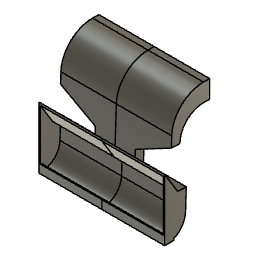
Goal_Chute (Autodesk Fusion 360 design; units mm, degrees)
Autodesk Fusion 360 part; units mm, degrees
note: some values were not read from the file. Set by a fixed rule: which sketch regions a step uses.
sketch "Sketch1" plane through (0, 0, 0) normal (0, 1, 0) x (1, 0, 0) in component "Front Board"
  line L0 (-457.2, -152.4) -> (457.2, -152.4)
  line L1 (457.2, -152.4) -> (457.2, 152.4)
  line L2 (457.2, 152.4) -> (-457.2, 152.4)
  line L3 (-457.2, 152.4) -> (-457.2, -152.4)
  line L4 (-127, -53.975) -> (127, -53.975)
  line L5 (127, -53.975) -> (127, 50.8)
  line L6 (127, 50.8) -> (-127, 50.8)
  line L7 (-127, 50.8) -> (-127, -53.975)
  dimension "d10" = 914.4
  dimension "d11" = 304.8
  dimension "d14" = 254
  dimension "d15" = 104.775
  dimension "d16" = 98.425
  dimension "d189" = 152.4
  dimension "d190" = 127
  dimension "d258" = 457.2
  constraint horizontal L0
  constraint vertical L1
  constraint horizontal L2
  constraint vertical L3
  constraint horizontal L4
  constraint vertical L5
  constraint horizontal L6
  constraint vertical L7
  measures "d10" distance of L0.start L0.end
  measures "d11" distance of L0.start L2.end
  measures "d14" distance of L4.start L4.end
  measures "d15" distance of L4.start L6.end
  measures "d16" distance of L0 L4
  measures "d189" distance of origin L0
  measures "d190" distance of origin L5
  measures "d258" distance of origin L3
extrude "Extrude1" add sketch "Sketch1" against normal blind 12.7 makes body 1 in component "Front Board"
sketch "Sketch1 (2)" plane through (0, 0, 0) normal (0, 1, 0) x (1, 0, 0) in component "Back Board"
  line L0 (457.2, -110.3312) -> (-457.2, -110.3312)
  line L1 (-457.2, -110.3312) -> (-457.2, 110.3312)
  line L2 (-457.2, 110.3312) -> (457.2, 110.3312)
  line L3 (457.2, 110.3312) -> (457.2, -110.3312)
  line L4 (114.3, -110.3312) -> (114.3, -89.6938)
  line L5 (114.3, -89.6938) -> (-114.3, -89.6938)
  line L6 (-114.3, -89.6938) -> (-114.3, -110.3312)
  dimension "d20" = 914.4
  dimension "d21" = 220.6625
  dimension "d22" = 110.3313
  dimension "d23" = 457.2
  dimension "d24" = 200.025
  dimension "d25" = 228.6
  dimension "d26" = 114.3
  constraint horizontal L0
  constraint vertical L1
  constraint horizontal L2
  constraint vertical L3
  constraint coincident L0 L4.start
  constraint perpendicular L0 L4
  constraint perpendicular L4 L5
  constraint coincident L0 L6.end
  constraint perpendicular L0 L6
  measures "d20" distance of L0.start L0.end
  measures "d21" distance of L0.start L2.end
  measures "d22" distance of origin L0
  measures "d23" distance of origin L3
  measures "d24" distance of L2 L5
  measures "d25" distance of L4.end L5.end
  measures "d26" distance of origin L4
extrude "Extrude1'" add sketch "Sketch1 (2)" against normal blind 12.7 separate body contours L0 L1 L2 L3 L4 L5 L6 makes body 2 in component "Back Board"
sketch "Sketch2" plane through (0, 0, 0) normal (1, 0, 0) x (0, 1, 0) in component "Chute"
  line L0 (0, -50.8) -> (2.54, -50.8)
  line L1 (2.54, -50.8) -> (2.54, -65.7225)
  arc A0 (2.54, -65.7225) -> (40.64, -28.8941) centre (2.5612, -27.6225) ccw
  line L2 (40.64, -28.8941) -> (44.45, 85.198)
  arc A1 (95.25, 134.3025) -> (44.45, 85.198) centre (95.2217, 83.5025) ccw
  line L3 (0, -50.8) -> (0, -68.2625)
  arc A2 (95.25, 166.0525) -> (32.4145, 105.3077) centre (95.2217, 103.2103) ccw
  arc A3 (2.54, -68.2625) -> (43.1786, -28.9789) centre (2.5612, -27.6225) ccw
  arc A4 (95.25, 131.7625) -> (46.9886, 85.1132) centre (95.2217, 83.5025) ccw
  line L4 (95.25, 134.3025) -> (95.25, 131.7625)
  line L5 (46.9886, 85.1132) -> (43.1786, -28.9789)
  line L6 (32.4145, 105.3077) -> (29.4039, 15.1538)
  line L7 (95.25, 166.0525) -> (95.25, 168.5925)
  arc A5 (95.25, 168.5925) -> (29.8759, 105.3924) centre (95.2217, 103.2103) ccw
  line L8 (0, 53.975) -> (0, 58.815)
  line L9 (29.8759, 105.3924) -> (26.8653, 15.2386)
  line L10 (46.9886, 85.1132) -> (44.45, 85.198)
  line L11 (31.7571, 85.6219) -> (29.2185, 85.7066)
  line L12 (31.7571, 85.6219) -> (44.45, 85.198)
  line L13 (95.25, 166.0525) -> (95.25, 134.3025)
  line L14 (0, 53.975) -> (0, -50.8)
  line L15 (95.25, 134.3025) -> (107.95, 134.3025)
  line L16 (107.95, 131.7625) -> (107.95, 134.3025)
  line L17 (95.25, 131.7625) -> (107.95, 131.7625)
  line L18 (95.25, 168.5925) -> (107.95, 168.5925)
  line L19 (107.95, 168.5925) -> (107.95, 166.0525)
  line L20 (107.95, 166.0525) -> (95.25, 166.0525)
  line L21 (92.71, 131.6971) -> (92.71, 168.5442)
  line L22 (42.012, 12.1914) -> (26.7805, 12.7)
  line L23 (42.012, 12.1914) -> (44.5506, 12.1066)
  line L24 (42.0968, 14.7299) -> (44.6354, 14.6452)
  line L25 (29.4039, 15.1538) -> (29.3191, 12.6152)
  line L26 (26.8653, 15.2386) -> (26.7805, 12.7)
  line L27 (42.0968, 14.7299) -> (29.4039, 15.1538)
  line L28 (26.8653, 15.2386) -> (29.4039, 15.1538)
  line L29 (0, 58.815) -> (26.8653, 15.2386)
  line L30 (26.7805, 12.7) -> (25.4184, 12.7455)
  line L31 (25.4184, 12.7455) -> (0, 53.975)
  line L32 (19.05, -61.9697) -> (19.05, -64.7672)
  line L33 (0, -68.2625) -> (2.54, -68.2625)
  line L34 (2.54, -68.2625) -> (19.05, -68.2625)
  line L35 (19.05, -68.2625) -> (19.05, -64.7672)
  line L36 (2.54, -65.7225) -> (0, -65.7225)
  line L37 (2.54, -65.7225) -> (19.05, -65.7225)
  line L38 (95.25, 144.4625) -> (92.71, 144.4625)
  line L39 (107.95, 166.0525) -> (107.95, 134.3025)
  point P0 (0, -50.8)
  point P1 (0, 53.975)
  point P2 (95.25, 131.7625)
  point P3 (107.95, 152.4)
  point P4 (95.25, -68.2625)
  dimension "d252" = 2.54
  dimension "d254" = 38.1
  dimension "d256" = 38.1
  dimension "d260" = 50.8
  dimension "d261" = 50.8
  dimension "d272" = 2.54
  dimension "d273" = 2.54
  dimension "d275" = 48.26
  dimension "d276" = 12.7
  dimension "d277" = 2.54
  dimension "d280" = 2.54
  dimension "d281" = 65.3822
  dimension "d282" = 62.8422
  dimension "d324" = 2.54
  dimension "d327" = 40.64
  dimension "d341" = 63.5
  dimension "d346" = 2.54
  dimension "d347" = 2.54
  dimension "d352" = 19.05
  dimension "d371" = 31.75
  dimension "d372" = 12.7
  constraint horizontal L0
  constraint perpendicular L0 L1
  constraint coincident P0 L0.start
  constraint tangent A0 L2
  constraint perpendicular L0 L3
  constraint tangent L2 A1
  constraint vertical A1.centre A2.centre
  constraint vertical L4
  constraint equal L2 L5
  constraint parallel L2 L5
  constraint tangent A4 L5
  constraint tangent A2 L6
  constraint parallel L2 L6
  constraint vertical L7
  constraint coincident P1 L8.start
  constraint vertical L8
  constraint parallel L6 L9
  constraint tangent A5 L9
  constraint tangent A3 L5
  constraint coincident L6 L11.start
  constraint coincident L9 L11.end
  constraint perpendicular L9 L11
  constraint collinear L10 L11
  constraint coincident L2 L22.start
  constraint coincident P2 A4.start
  constraint perpendicular L13 L15
  constraint perpendicular L16 L17
  constraint perpendicular L15 L16
  constraint perpendicular L18 L19
  constraint perpendicular L19 L20
  constraint perpendicular L7 L18
  constraint coincident A2.start L7.start
  constraint vertical L15.end L18.end
  constraint coincident A4 L21.start
  constraint coincident A5 L21.end
  constraint vertical L21
  constraint coincident L2 L24.start
  constraint coincident L9.end L26.start
  constraint coincident L5 L23.end
  constraint coincident L5 L24.end
  constraint coincident L22 L26.end
  constraint parallel L9 L26
  constraint parallel L6 L25
  constraint coincident L22 L25.end
  constraint parallel L22 L23
  constraint parallel L27 L28
  constraint parallel L24 L27
  constraint parallel L29 L31
  constraint parallel L22 L30
  constraint perpendicular L2 L22
  constraint parallel L22 L27
  constraint coincident A0 L32.start
  constraint coincident A3 L32.end
  constraint vertical L32
  constraint perpendicular L3 L33
  constraint vertical L1.end A3.start
  constraint coincident A3.start L33.end
  constraint horizontal L34
  constraint vertical L35
  constraint horizontal L3.end P4
  constraint coincident L3 L36.end
  constraint perpendicular L3 L36
  constraint coincident L32 L37.end
  constraint perpendicular L1 L37
  constraint vertical L19.end P3
  constraint coincident L13 L38.start
  constraint coincident L21 L38.end
  constraint perpendicular L21 L38
  measures "d252" distance of P0 L0.end
  measures "d254" radius of A0
  measures "d256" horizontal distance of L1.end A0.end
  measures "d260" radius of A1
  measures "d261" horizontal distance of A1.start L2.end
  measures "d272" distance of A1.start P2
  measures "d273" distance of L2 L5
  measures "d275" radius of A4
  measures "d276" distance of L2 L6
  measures "d277" distance of A2.start L7.end
  measures "d280" distance of L6 L9
  measures "d281" radius of A5
  measures "d282" radius of A2
  measures "d324" distance of L13 L21
  measures "d327" radius of A3
  measures "d341" vertical distance of P0 L22.end
  measures "d346" distance of L29 L31
  measures "d347" distance of L22 L27
  measures "d352" distance of L3 L32
  measures "d371" distance of L15.end L19.end
  measures "d372" distance of P2 L38.start
extrude "Extrude3" add sketch "Sketch2" along normal blind 2.54 separate body contours A2 L6 A5 L9 L11 L21 | A1 A2 L6 L12 L21 | A2 L7 A5 L21 | A1 A4 L10 L21 | L7 L18 L19 L20 | A2 L13 L21 L38 | A1 L13 L21 L38 | A1 A4 L4 L21 | L13 L15 L20 L39 | L4 L15 L16 L17 makes body 3 in component "Chute"
extrude "Extrude4" add sketch "Sketch2" along normal blind 114.3 contours A2 L6 A5 L9 L11 L21 | A2 L7 A5 L21 | A1 A4 L10 L21 | L7 L18 L19 L20 | A1 A4 L4 L21 | L4 L15 L16 L17 bodies 3 in component "Chute"
extrude "Extrude5" add sketch "Sketch2" against normal blind 2.54 from surface at -12.7 separate body contours A0 A3 L32 L37 | L0 L1 A0 L2 L14 L22 L30 L31 | L0 L1 L3 L36 | L3 A3 L33 L36 L37 | L8 L26 L29 L30 L31 | A0 L2 A3 L5 L23 L32 | L22 L25 L26 L28 | L2 L22 L25 L27 | L2 L5 L23 L24 makes body 4 in component "Chute"
extrude "Extrude6" add sketch "Sketch2" along normal blind 88.9 from surface at -12.7 contours A0 A3 L32 L37 | L0 L1 L3 L36 | L3 A3 L33 L36 L37 | L8 L26 L29 L30 L31 | A0 L2 A3 L5 L23 L32 | L22 L25 L26 L28 | L2 L22 L25 L27 | L2 L5 L23 L24 bodies 4 in component "Chute"
extrude "Extrude7" add sketch "Sketch2" along normal blind 38.1 from surface at 76.2 contours A0 A3 L32 L37 | L0 L1 L3 L36 | L3 A3 L33 L36 L37 | L8 L26 L29 L30 L31 | A0 L2 A3 L5 L23 L32 | L22 L25 L26 L28 | L2 L5 L23 L24 bodies 4 in component "Chute"
extrude "Extrude24" add sketch "Sketch2" along normal blind 10.16 and the other way blind 15.24 contours A3 L34 L35 L37 | A3 L35 L37 bodies 4 in component "Chute"
ref_plane "WorkPlane1" through (-15.24, 44.6354, 14.6452) normal (0, 0.999443, -0.033375) x (-1, 0, 0) in component "Chute"
sketch "Sketch3" plane through (0, 44.0971, -1.4726) normal (0, 0.999443, -0.033375) x (-1, 0, 0) in component "Chute"
  line L0 (-3.175, 86.6341) -> (-76.2, 48.5341)
  line L1 (-76.2, 48.5341) -> (-76.2, 16.1267)
  line L2 (-114.3, 86.6341) -> (-3.175, 86.6341)
  line L3 (-114.3, 86.6341) -> (-114.3, 16.1267)
  line L4 (-114.3, 16.1267) -> (-76.2, 16.1267)
  line L5 (-76.2, 16.1267) -> (-73.025, 16.1267)
  line L6 (-73.025, 16.1267) -> (-73.025, 46.6094)
  line L7 (0, 84.7094) -> (-73.025, 46.6094)
  line L8 (-3.175, 86.6341) -> (0, 86.6341)
  line L9 (0, 84.7094) -> (0, 86.6341)
  point P0 (-114.3, 86.6341)
  point P1 (-114.3, 16.1267)
  dimension "d294" = 38.1
  dimension "d295" = 38.1
  dimension "d296" = 111.125
  dimension "d297" = 3.175
  dimension "d300" = 3.175
  dimension "d301" = 3.175
  constraint vertical L1
  constraint horizontal L2
  constraint horizontal L4
  constraint vertical L3
  constraint coincident P0 L2.start
  constraint horizontal L5
  constraint perpendicular L5 L6
  constraint parallel L0 L7
  constraint parallel L2 L8
  constraint perpendicular L8 L9
  constraint coincident P1 L3.end
  measures "d294" vertical distance of L0.end L0.start
  measures "d295" distance of L1.end P1
  measures "d296" distance of P0 L0.start
  measures "d297" distance of L1.end L5.end
  measures "d300" horizontal distance of L0.start L7.start
  measures "d301" distance of L0 L7
extrude "Extrude8" add sketch "Sketch3" against normal blind 17.78 bodies 4 3 in component "Chute"
extrude "Extrude17" cut sketch "Sketch3" against normal blind 12.7 from surface at -2.54 contours L0 L1 L2 L3 L4 bodies 4 in component "Chute"
mirror "MirrorComponent7" about plane through (0, 0, 0) normal (0, 0, 1) of bodies 4 makes body 5 in component "Chute(Mirror)"
component "Front Board" placed x (1, 0, 0) y (0, 1, 0) z (0, 0, 1) at (0, 0, 0)
component "Back Board" placed x (1, 0, 0) y (0, 1, 0) z (0, 0, 1) at (0, 107.95, 42.0688)
component "Chute" placed x (1, 0, 0) y (0, 1, 0) z (0, 0, 1) at (-114.3, 0, 0)
component "Chute(Mirror)" placed x (-1, 0, 0) y (0, 1, 0) z (0, 0, -1) at (114.3, 0, 0)
equation "d21 = 8 in + ( ( 11 / 16 ) * 1 in )"
equation "d22 = d21 / 2"
equation "d23 = d20 / 2"
equation "d26 = d25 / 2"
equation "d32 = 3 in + ( 3 / 4 ) * 1 in"
equation "d55 = d63 + 0.375 in"
equation "d63 = 2 in"
equation "d190 = d14 / 2"
equation "d252 = d272"
equation "d258 = d10 / 2"
equation "d261 = d260"
equation "d273 = d272"
equation "d275 = d260 - d272"
equation "d277 = d272"
equation "d280 = d272"
equation "d281 = d282 + d272"
equation "d300 = d297"
equation "d301 = d297"
equation "d324 = d272"
equation "d327 = d254 + d272"
equation "d346 = d272"
equation "d347 = d272"
